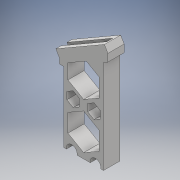
# Autodesk Inventor part: Screen Docking Reciever
Saved by Autodesk Inventor 2018 (Build 220112000, 112)
## iProperties
Created: 2018-05-10
Part Number: Screen Docking Reciever
Material: Generic
Document SubType Name: Modeling
Designer: Jasper
Density: 1 g/cm^3
Appearance: Default
Author: Jasper
Autodesk Inventor part; units mm, degrees
ref_plane "YZ Plane" through (0, 0, 0) normal (1, 0, 0) x (0, 1, 0)
ref_plane "XZ Plane" through (0, 0, 0) normal (0, 1, 0) x (-1, 0, 0)
ref_plane "XY Plane" through (0, 0, 0) normal (0, 0, 1) x (1, 0, 0)
sketch "Sketch1" plane through (0, 0, 0) normal (0, 1, 0) x (-1, 0, 0)
  line L0 (-22.5, 35) -> (22.5, 35)
  line L1 (22.5, 35) -> (22.5, -35)
  line L2 (22.5, -35) -> (-22.5, -35) construction
  line L3 (-22.5, -35) -> (-22.5, 35)
  line L4 (-22.5, 35) -> (22.5, -35) construction
  line L5 (22.5, 35) -> (-22.5, -35) construction
  line L6 (22.5, -34) -> (-22.5, -34) construction
  circle A0 centre (11, -34) radius 5
  line L7 (0, 0) -> (0, -35) construction
  circle A1 centre (-11, -34) radius 5
  line L8 (22.5, 35) -> (-22.5, 60.9808)
  line L9 (-22.5, 60.9808) -> (-22.5, 35)
  line L10 (22.5, -35) -> (15.899, -35)
  line L11 (6.101, -35) -> (-6.101, -35)
  line L12 (-15.899, -35) -> (-22.5, -35)
  dimension "d0" = 45
  dimension "d1" = 70
  dimension "d2" = 1
  dimension "d3" = 10
  dimension "d4" = 11
  dimension "d6" = 30
  constraints: 26 end point, 7 point on line, 4 point on circle, 3 midpoint, 2 centre point, 2 parallel, 2 perpendicular, 1 collinear, 1 horizontal, 1 symmetric about line, 1 vertical, 1 other
  measures "d0" distance of L1.end L2.end
  measures "d1" distance of L0.end L1.end
  measures "d2" distance between parallel lines of L2 L6
  measures "d3" diameter of A0
  measures "d4" distance from line of L7 A0.centre
  measures "d6" angle of L8 L0
extrude "Extrusion1" add sketch "Sketch1" along normal blind 15 contours L9 L8 L0 | L0 L1 L10 A0 L11 A1 L12 L3
sketch "Sketch2" plane through (0, 15, 0) normal (0, 1, 0) x (1, 0, 0)
  line L0 (-22.5, -35) -> (-22.5, -30)
  line L1 (-22.5, -30) -> (-18.5, -30)
  line L2 (-18.5, -30) -> (-18.5, 35)
  line L3 (-15.899, 35) -> (-22.5, 35) projected
  line L4 (-22.5, 35) -> (-22.5, -30)
  line L5 (-22.5, -35) -> (22.5, -60.9808) projected
  line L6 (22.5, -60.9808) -> (22.5, 35) projected
  line L7 (22.5, -60.9808) -> (22.5, -53.9808)
  line L8 (22.5, -53.9808) -> (18.5, -51.6714)
  line L9 (18.5, -51.6714) -> (18.5, 35)
  line L10 (18.5, 35) -> (22.5, 35)
  line L11 (0, 34.5774) -> (18.5, 23.8964) construction
  line L12 (18.5, 23.8964) -> (18.5, 2.5344) construction
  line L13 (18.5, 2.5344) -> (0, -8.1466) construction
  line L14 (0, -8.1466) -> (-18.5, 2.5344) construction
  line L15 (-18.5, 2.5344) -> (-18.5, 23.8964) construction
  line L16 (-18.5, 23.8964) -> (0, 34.5774) construction
  arc A0 (-15.899, 35) -> (-6.101, 35) centre (-11, 34) ccw construction
  arc A1 (6.101, 35) -> (15.899, 35) centre (11, 34) ccw construction
  line L17 (-14.5, 4.8438) -> (0, -3.5278)
  line L18 (0, -3.5278) -> (14.5, 4.8438)
  line L19 (14.5, 4.8438) -> (14.5, 21.587)
  line L20 (14.5, 21.587) -> (0, 29.9585)
  line L21 (0, 29.9585) -> (-14.5, 21.587)
  line L22 (-14.5, 21.587) -> (-14.5, 4.8438)
  line L23 (0, -8.1466) -> (-18.5, -8.1466) construction
  line L24 (-14.5, -21.137) -> (0, -12.7654)
  line L25 (0, -12.7654) -> (14.5, -21.137)
  line L26 (14.5, -21.137) -> (14.5, -37.8801)
  line L27 (14.5, -37.8801) -> (0, -46.2517)
  line L28 (0, -46.2517) -> (-14.5, -37.8801) construction
  line L29 (-14.5, -37.8801) -> (-14.5, -21.137)
  line L30 (-15.5, -4.7787) -> (-9.6667, -1.4108)
  line L31 (-9.6667, -1.4108) -> (-3.8333, -4.7787)
  line L32 (-3.8333, -4.7787) -> (-3.8333, -11.5144)
  line L33 (-3.8333, -11.5144) -> (-9.6667, -14.8823)
  line L34 (-9.6667, -14.8823) -> (-15.5, -11.5144)
  line L35 (-15.5, -11.5144) -> (-15.5, -4.7787)
  line L36 (0, -8.1466) -> (0, -47.9904) construction
  line L37 (-22.5, -35) -> (22.5, -60.9808) construction
  line L38 (15.5, -4.7787) -> (9.6667, -1.4108)
  line L39 (9.6667, -1.4108) -> (3.8333, -4.7787)
  line L40 (3.8333, -4.7787) -> (3.8333, -11.5144)
  line L41 (3.8333, -11.5144) -> (9.6667, -14.8823)
  line L42 (9.6667, -14.8823) -> (15.5, -11.5144)
  line L43 (15.5, -11.5144) -> (15.5, -4.7787)
  line L44 (2.4942, -44.8116) -> (-14.5, -35)
  point P0 (0, 0)
  point P1 (0, 13.2154)
  point P2 (-9.6667, -8.1466)
  dimension "d9" = 5
  dimension "d10" = 4
  dimension "d11" = 7
  dimension "d12" = 60
  dimension "d13" = 4
  dimension "d14" = 4
  dimension "d15" = 3
  dimension "d16" = 3
  dimension "d17" = 4
  constraints: 82 end point, 12 symmetric about line, 7 point on line, 4 parallel, 4 perpendicular, 2 tangent, 2 vertical, 1 collinear, 1 midpoint, 31 other
  measures "d9" distance of L0.start L0.end
  measures "d10" distance of L0.end L1.end
  measures "d11" distance of L5.end L7.end
  measures "d12" angle of L6 L8
  measures "d13" horizontal distance of L7.end L8.end
  measures "d14" distance between parallel lines of L14 L17
  measures "d15" distance between parallel lines of L24 L33
  measures "d16" distance between parallel lines of L35 L2
  measures "d17" distance between parallel lines of L5 L44
extrude "Extrusion2" cut sketch "Sketch2" against normal through all
sketch "Sketch3" plane through (22.5, 0, 60.9808) normal (-0.5, 0, 0.8660254) x (0.8660254, 0, 0.5)
  line L0 (-51.9615, 0) -> (-51.9615, 15) projected
  line L1 (-51.9615, 15) -> (0, 15) projected
  line L2 (-39.8405, 15) -> (-48.2121, 15) projected
  line L3 (-51.9615, 0) -> (0, 0) projected
  line L4 (0, 0) -> (0, 15) projected
  line L5 (-51.9615, 15) -> (0, 15) projected
  line L6 (-51.9615, 0) -> (-51.9615, 15) projected
  line L7 (-51.9615, 7.5) -> (0, 7.5) construction
  line L8 (0, 2.25) -> (-51.9615, 2.25)
  line L9 (-51.9615, 2.25) -> (-51.9615, 12.75)
  line L10 (-51.9615, 12.75) -> (0, 12.75)
  line L11 (0, 12.75) -> (0, 2.25)
  line L12 (0, 2.25) -> (-51.9615, 12.75) construction
  line L13 (-51.9615, 2.25) -> (0, 12.75) construction
  line L14 (-3, 2.25) -> (-3, 12.75)
  point P0 (-49.976, 0)
  point P1 (-25.9808, 7.5)
  dimension "d20" = 10.5
  dimension "d21" = 3
  constraints: 16 end point, 5 midpoint, 3 point on line, 2 parallel, 2 perpendicular, 1 horizontal
  measures "d20" distance between parallel lines of L10 L8
  measures "d21" distance between parallel lines of L4 L14
extrude "Extrusion3" add sketch "Sketch3" along normal blind 3.2 contours L0 L8 L4 L3 | L0 L1 L4 L10 | L14 L10 L4 L8
sketch "Sketch5" plane through (20.9, 0, 63.752) normal (-0.5, 0, 0.8660254) x (0.8660254, 0, 0.5)
  line L0 (-51.9615, 0) -> (0, 0) projected
  line L1 (-51.9615, 2.25) -> (-51.9615, 12.75) projected
  line L2 (-51.9615, 2.25) -> (-51.9615, 0) projected
  line L3 (-51.9615, 15) -> (-51.9615, 12.75) projected
  line L4 (0, 15) -> (-51.9615, 15) projected
  line L5 (-3, 12.75) -> (-3, 2.25) projected
  line L6 (0, 0) -> (0, 15) projected
  line L7 (-51.9615, 7.5) -> (0, 7.5) construction
  line L8 (-51.9615, 4.75) -> (0, 4.75)
  line L9 (0, 4.75) -> (0, 10.25)
  line L10 (0, 10.25) -> (-51.9615, 10.25)
  line L11 (-51.9615, 10.25) -> (-51.9615, 4.75)
  line L12 (-51.9615, 4.75) -> (0, 10.25) construction
  line L13 (0, 4.75) -> (-51.9615, 10.25) construction
  line L14 (-3, 4.75) -> (-3, 10.25)
  point P0 (-49.976, 0)
  point P1 (-25.9808, 7.5)
  dimension "d24" = 5.5
  constraints: 16 end point, 5 midpoint, 5 point on line, 2 parallel, 1 horizontal, 1 perpendicular
  measures "d24" distance between parallel lines of L10 L8
extrude "Extrusion4" add sketch "Sketch5" along normal blind 3.2 contours L2 L1 L8 L6 L0 | L8 L5 L10 L6 | L10 L1 L3 L4 L6
sketch "Sketch6" plane through (19.9019, 2.25, 59.4808) normal (-0.5, 0, 0.8660254) x (0.8660254, 0, 0.5)
  line L0 (0, 8) -> (0, 2.5) projected
  line L1 (-48.9615, 0) -> (-48.9615, 10.5) projected
  line L2 (0, 5.25) -> (-32.25, 5.25) construction
  circle A0 centre (-32.25, 5.25) radius 1.5
  point P0 (-46.976, -2.25)
  dimension "d27" = 32.25
  dimension "d28" = 3
  constraints: 2 end point, 1 centre point, 1 coincident, 1 horizontal, 1 midpoint
  measures "d27" distance of L2.start L2.end
  measures "d28" diameter of A0
extrude "Extrusion5" cut sketch "Sketch6" against normal blind 3.2
fillet "Fillet1" radius 2 1 edges at (-9.3264, 7.5, 42.6058)
body "Solid1"
